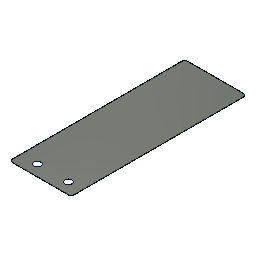
sofle_v2_oled_cover_0.1 (Autodesk Fusion 360 design; units mm, degrees)
Autodesk Fusion 360 part; units mm, degrees
note: some values were not read from the file. Set by a fixed rule: which sketch regions a step uses.
sketch "Sketch1" plane through (0, 0, 0) normal (0, 1, 0) x (1, 0, 0)
  line L0 (8.95, 28.225) -> (-8.95, 28.225)
  line L1 (-9.95, 27.225) -> (-9.95, -27.225)
  line L2 (-8.95, -28.225) -> (8.95, -28.225)
  line L3 (9.95, -27.225) -> (9.95, 27.225)
  line L4 (9.95, 28.225) -> (-9.95, -28.225) construction
  line L5 (-9.95, 28.225) -> (9.95, -28.225) construction
  arc A0 (-9.95, -27.225) -> (-8.95, -28.225) centre (-8.95, -27.225) ccw
  arc A1 (8.95, -28.225) -> (9.95, -27.225) centre (8.95, -27.225) ccw
  arc A2 (-8.95, 28.225) -> (-9.95, 27.225) centre (-8.95, 27.225) ccw
  arc A3 (9.95, 27.225) -> (8.95, 28.225) centre (8.95, 27.225) ccw
  dimension "d1" = 19.9
  dimension "d2" = 56.45
  dimension "d3" = 1
  dimension "d4" = 1
  dimension "d5" = 1
  dimension "d6" = 1
  constraint horizontal L0
  constraint perpendicular L0 L1
  constraint parallel L0 L2
  constraint parallel L1 L3
  constraint coincident L4 origin
  constraint coincident L5 origin
  constraint coincident L4.end L2
  constraint coincident L4.end L1
  constraint tangent L2 A0
  constraint tangent L1 A0
  constraint coincident L5.end L2
  constraint coincident L5.end L3
  constraint tangent L2 A1
  constraint tangent L3 A1
  constraint coincident L5.start L1
  constraint coincident L5.start L0
  constraint tangent L1 A2
  constraint tangent L0 A2
  constraint coincident L4.start L0
  constraint coincident L4.start L3
  constraint tangent L0 A3
  constraint tangent L3 A3
  measures "d1" distance of L4.end L5.end
  measures "d2" distance of L5.start L4.end
  measures "d3" radius of A0
  measures "d4" radius of A1
  measures "d5" radius of A2
  measures "d6" radius of A3
extrude "Extrude1" add sketch "Sketch1" along normal blind 0.1
sketch "Sketch2" plane through (0, 0.1, 0) normal (0, 1, 0) x (-1, 0, 0)
  arc A0 (-9.95, -27.225) -> (-8.95, -28.225) centre (-8.95, -27.225) ccw
  line L0 (-8.95, -28.225) -> (8.95, -28.225)
  arc A1 (8.95, -28.225) -> (9.95, -27.225) centre (8.95, -27.225) ccw
  line L1 (9.95, -27.225) -> (9.95, 27.225)
  arc A2 (9.95, 27.225) -> (8.95, 28.225) centre (8.95, 27.225) ccw
  line L2 (8.95, 28.225) -> (-8.95, 28.225)
  arc A3 (-8.95, 28.225) -> (-9.95, 27.225) centre (-8.95, 27.225) ccw
  line L3 (-9.95, 27.225) -> (-9.95, -27.225)
  line L4 (0, 28.225) -> (0, 24.625)
  line L5 (0, 24.625) -> (9.95, 24.625)
  line L6 (0, 24.625) -> (-9.95, 24.625)
  line L7 (9.95, 24.625) -> (4.55, 24.625)
  circle A4 centre (4.55, 24.625) radius 1.125
  line L8 (4.55, 24.625) -> (-5.45, 24.625)
  circle A5 centre (-5.45, 24.625) radius 1.125
  dimension "d9" = 3.6
  dimension "d10" = 5.4
  dimension "d11" = 2.25
  dimension "d12" = 10
  dimension "d13" = 2.25
  constraint midpoint L2 L4.start
  constraint perpendicular L2 L4
  constraint coincident L1 L5.end
  constraint perpendicular L1 L5
  constraint coincident L3 L6.end
  constraint perpendicular L3 L6
  constraint perpendicular L1 L7
  constraint coincident L7.end A4.centre
  constraint coincident L6 L8.end
  constraint coincident L8.end A5.centre
  measures "d9" distance of L4.start L4.end
  measures "d10" distance of L5.end L7.end
  measures "d11" diameter of A4
  measures "d12" distance of L7.end L8.end
  measures "d13" diameter of A5
extrude "Extrude2" cut sketch "Sketch2" against normal blind 0.1 contours L6 L8 A5 | L6 L8 A5 | L5 L7 A4 L8 | L5 L7 A4 L8
sketch "Sketch3" plane through (0, 0.1, 0) normal (0, 1, 0) x (-1, 0, 0)
  circle A0 centre (4.55, 24.625) radius 1.125
  circle A1 centre (-5.45, 24.625) radius 1.125
  arc A2 (-9.95, -27.225) -> (-8.95, -28.225) centre (-8.95, -27.225) ccw
  line L0 (-8.95, -28.225) -> (8.95, -28.225)
  arc A3 (8.95, -28.225) -> (9.95, -27.225) centre (8.95, -27.225) ccw
  line L1 (9.95, -27.225) -> (9.95, 27.225)
  arc A4 (9.95, 27.225) -> (8.95, 28.225) centre (8.95, 27.225) ccw
  line L2 (8.95, 28.225) -> (-8.95, 28.225)
  arc A5 (-8.95, 28.225) -> (-9.95, 27.225) centre (-8.95, 27.225) ccw
  line L3 (-9.95, 27.225) -> (-9.95, -27.225)
